Autodesk Fusion 360 part; units mm, degrees
(part 10 of 40)
  spline S57 degree 5 poles (181.0205, 97.4897) (181.0048, 97.4632) (180.9726, 97.4105) (180.9223, 97.3328) (180.8513, 97.2319) (180.7572, 97.1094) (180.6593, 96.9894) (180.5591, 96.8711) (180.4576, 96.7536) (180.3553, 96.6366) (180.252, 96.5203) (180.1476, 96.4049) (180.0417, 96.2906) (179.9339, 96.1776) (179.8243, 96.066) (179.713, 95.9556) (179.6004, 95.8463) (179.4865, 95.7378) (179.3717, 95.6302) (179.256, 95.5233) (179.1393, 95.4172) (179.0215, 95.3119) (178.9028, 95.2074) (178.7829, 95.1039) (178.662, 95.0012) (178.5401, 94.8993) (178.4172, 94.7983) (178.2934, 94.698) (178.1687, 94.5985) (178.0432, 94.4997) (177.9169, 94.4016) (177.7897, 94.3043) (177.6617, 94.2077) (177.5329, 94.1119) (177.4032, 94.0168) (177.2728, 93.9224) (177.1415, 93.8288) (177.0096, 93.7358) (176.8768, 93.6436) (176.7434, 93.552) (176.6092, 93.4612) (176.4743, 93.371) (176.3387, 93.2815) (176.2025, 93.1927) (176.0655, 93.1045) (175.9278, 93.0171) (175.7895, 92.9303) (175.6505, 92.8442) (175.5109, 92.7587) (175.3706, 92.6739) (175.2297, 92.5898) (175.0882, 92.5063) (174.946, 92.4235) (174.8032, 92.3413) (174.6599, 92.2597) (174.5159, 92.1788) (174.3713, 92.0986) (174.2262, 92.019) (174.0805, 91.94) (173.9342, 91.8617) (173.7873, 91.784) (173.6399, 91.7069) (173.4919, 91.6305) (173.3434, 91.5547) (173.1943, 91.4795) (173.0447, 91.405) (172.8946, 91.331) (172.7439, 91.2577) (172.5927, 91.1851) (172.4411, 91.113) (172.2889, 91.0416) (172.1667, 90.9849) (172.0748, 90.9427) (172.0135, 90.9147) (171.9828, 90.9007) knots 0 0 0 0 0 0 0.01428571 0.02857143 0.04285714 0.05714286 0.07142857 0.08571429 0.1 0.11428571 0.12857143 0.14285714 0.15714286 0.17142857 0.18571429 0.2 0.21428571 0.22857143 0.24285714 0.25714286 0.27142857 0.28571429 0.3 0.31428571 0.32857143 0.34285714 0.35714286 0.37142857 0.38571429 0.4 0.41428571 0.42857143 0.44285714 0.45714286 0.47142857 0.48571429 0.5 0.51428571 0.52857143 0.54285714 0.55714286 0.57142857 0.58571429 0.6 0.61428571 0.62857143 0.64285714 0.65714286 0.67142857 0.68571429 0.7 0.71428571 0.72857143 0.74285714 0.75714286 0.77142857 0.78571429 0.8 0.81428571 0.82857143 0.84285714 0.85714286 0.87142857 0.88571429 0.9 0.91428571 0.92857143 0.94285714 0.95714286 0.97142857 0.98571429 1 1 1 1 1 1
  line L4287 (181.0205, 97.4897) -> (181.0048, 97.4632) construction
  line L4288 (181.0048, 97.4632) -> (180.9726, 97.4105) construction
  line L4289 (180.9726, 97.4105) -> (180.9223, 97.3328) construction
  line L4290 (180.9223, 97.3328) -> (180.8513, 97.2319) construction
  line L4291 (180.8513, 97.2319) -> (180.7572, 97.1094) construction
  line L4292 (180.7572, 97.1094) -> (180.6593, 96.9894) construction
  line L4293 (180.6593, 96.9894) -> (180.5591, 96.8711) construction
  line L4294 (180.5591, 96.8711) -> (180.4576, 96.7536) construction
  line L4295 (180.4576, 96.7536) -> (180.3553, 96.6366) construction
  line L4296 (180.3553, 96.6366) -> (180.252, 96.5203) construction
  line L4297 (180.252, 96.5203) -> (180.1476, 96.4049) construction
  line L4298 (180.1476, 96.4049) -> (180.0417, 96.2906) construction
  line L4299 (180.0417, 96.2906) -> (179.9339, 96.1776) construction
  line L4300 (179.9339, 96.1776) -> (179.8243, 96.066) construction
  line L4301 (179.8243, 96.066) -> (179.713, 95.9556) construction
  line L4302 (179.713, 95.9556) -> (179.6004, 95.8463) construction
  line L4303 (179.6004, 95.8463) -> (179.4865, 95.7378) construction
  line L4304 (179.4865, 95.7378) -> (179.3717, 95.6302) construction
  line L4305 (179.3717, 95.6302) -> (179.256, 95.5233) construction
  line L4306 (179.256, 95.5233) -> (179.1393, 95.4172) construction
  line L4307 (179.1393, 95.4172) -> (179.0215, 95.3119) construction
  line L4308 (179.0215, 95.3119) -> (178.9028, 95.2074) construction
  line L4309 (178.9028, 95.2074) -> (178.7829, 95.1039) construction
  line L4310 (178.7829, 95.1039) -> (178.662, 95.0012) construction
  line L4311 (178.662, 95.0012) -> (178.5401, 94.8993) construction
  line L4312 (178.5401, 94.8993) -> (178.4172, 94.7983) construction
  line L4313 (178.4172, 94.7983) -> (178.2934, 94.698) construction
  line L4314 (178.2934, 94.698) -> (178.1687, 94.5985) construction
  line L4315 (178.1687, 94.5985) -> (178.0432, 94.4997) construction
  line L4316 (178.0432, 94.4997) -> (177.9169, 94.4016) construction
  line L4317 (177.9169, 94.4016) -> (177.7897, 94.3043) construction
  line L4318 (177.7897, 94.3043) -> (177.6617, 94.2077) construction
  line L4319 (177.6617, 94.2077) -> (177.5329, 94.1119) construction
  line L4320 (177.5329, 94.1119) -> (177.4032, 94.0168) construction
  line L4321 (177.4032, 94.0168) -> (177.2728, 93.9224) construction
  line L4322 (177.2728, 93.9224) -> (177.1415, 93.8288) construction
  line L4323 (177.1415, 93.8288) -> (177.0096, 93.7358) construction
  line L4324 (177.0096, 93.7358) -> (176.8768, 93.6436) construction
  line L4325 (176.8768, 93.6436) -> (176.7434, 93.552) construction
  line L4326 (176.7434, 93.552) -> (176.6092, 93.4612) construction
  line L4327 (176.6092, 93.4612) -> (176.4743, 93.371) construction
  line L4328 (176.4743, 93.371) -> (176.3387, 93.2815) construction
  line L4329 (176.3387, 93.2815) -> (176.2025, 93.1927) construction
  line L4330 (176.2025, 93.1927) -> (176.0655, 93.1045) construction
  line L4331 (176.0655, 93.1045) -> (175.9278, 93.0171) construction
  line L4332 (175.9278, 93.0171) -> (175.7895, 92.9303) construction
  line L4333 (175.7895, 92.9303) -> (175.6505, 92.8442) construction
  line L4334 (175.6505, 92.8442) -> (175.5109, 92.7587) construction
  line L4335 (175.5109, 92.7587) -> (175.3706, 92.6739) construction
  line L4336 (175.3706, 92.6739) -> (175.2297, 92.5898) construction
  line L4337 (175.2297, 92.5898) -> (175.0882, 92.5063) construction
  line L4338 (175.0882, 92.5063) -> (174.946, 92.4235) construction
  line L4339 (174.946, 92.4235) -> (174.8032, 92.3413) construction
  line L4340 (174.8032, 92.3413) -> (174.6599, 92.2597) construction
  line L4341 (174.6599, 92.2597) -> (174.5159, 92.1788) construction
  line L4342 (174.5159, 92.1788) -> (174.3713, 92.0986) construction
  line L4343 (174.3713, 92.0986) -> (174.2262, 92.019) construction
  line L4344 (174.2262, 92.019) -> (174.0805, 91.94) construction
  line L4345 (174.0805, 91.94) -> (173.9342, 91.8617) construction
  line L4346 (173.9342, 91.8617) -> (173.7873, 91.784) construction
  line L4347 (173.7873, 91.784) -> (173.6399, 91.7069) construction
  line L4348 (173.6399, 91.7069) -> (173.4919, 91.6305) construction
  line L4349 (173.4919, 91.6305) -> (173.3434, 91.5547) construction
  line L4350 (173.3434, 91.5547) -> (173.1943, 91.4795) construction
  line L4351 (173.1943, 91.4795) -> (173.0447, 91.405) construction
  line L4352 (173.0447, 91.405) -> (172.8946, 91.331) construction
  line L4353 (172.8946, 91.331) -> (172.7439, 91.2577) construction
  line L4354 (172.7439, 91.2577) -> (172.5927, 91.1851) construction
  line L4355 (172.5927, 91.1851) -> (172.4411, 91.113) construction
  line L4356 (172.4411, 91.113) -> (172.2889, 91.0416) construction
  line L4357 (172.2889, 91.0416) -> (172.1667, 90.9849) construction
  line L4358 (172.1667, 90.9849) -> (172.0748, 90.9427) construction
  line L4359 (172.0748, 90.9427) -> (172.0135, 90.9147) construction
  line L4360 (172.0135, 90.9147) -> (171.9828, 90.9007) construction
  spline S58 degree 5 poles (171.8057, 104.1847) (171.7853, 104.1615) (171.7452, 104.1146) (171.6869, 104.0427) (171.6128, 103.944) (171.5254, 103.8167) (171.4416, 103.6865) (171.36, 103.5546) (171.2796, 103.4218) (171.2, 103.2883) (171.1213, 103.1542) (171.0437, 103.0193) (170.9678, 102.8832) (170.8937, 102.7457) (170.8214, 102.607) (170.7507, 102.4671) (170.6816, 102.3262) (170.6136, 102.1844) (170.5467, 102.0419) (170.4808, 101.8988) (170.416, 101.755) (170.3522, 101.6105) (170.2896, 101.4653) (170.2281, 101.3193) (170.1678, 101.1726) (170.1086, 101.0251) (170.0505, 100.877) (169.9934, 100.7283) (169.9373, 100.579) (169.8821, 100.4291) (169.8279, 100.2786) (169.7746, 100.1276) (169.7223, 99.976) (169.671, 99.8239) (169.6206, 99.6712) (169.5712, 99.518) (169.5226, 99.3642) (169.475, 99.21) (169.4283, 99.0553) (169.3825, 98.9001) (169.3375, 98.7444) (169.2934, 98.5882) (169.2502, 98.4316) (169.2079, 98.2745) (169.1664, 98.117) (169.1257, 97.9591) (169.0859, 97.8007) (169.047, 97.6419) (169.0089, 97.4827) (168.9716, 97.3231) (168.9351, 97.1631) (168.8994, 97.0027) (168.8646, 96.8419) (168.8305, 96.6807) (168.7973, 96.5191) (168.7648, 96.3572) (168.7332, 96.1949) (168.7023, 96.0323) (168.6723, 95.8693) (168.643, 95.706) (168.6145, 95.5423) (168.5867, 95.3783) (168.5597, 95.2139) (168.5336, 95.0492) (168.5081, 94.8842) (168.4834, 94.7189) (168.4595, 94.5533) (168.4364, 94.3874) (168.414, 94.2211) (168.3923, 94.0546) (168.3714, 93.8878) (168.3553, 93.7541) (168.3435, 93.6537) (168.3358, 93.5867) (168.332, 93.5531) knots 0 0 0 0 0 0 0.01428571 0.02857143 0.04285714 0.05714286 0.07142857 0.08571429 0.1 0.11428571 0.12857143 0.14285714 0.15714286 0.17142857 0.18571429 0.2 0.21428571 0.22857143 0.24285714 0.25714286 0.27142857 0.28571429 0.3 0.31428571 0.32857143 0.34285714 0.35714286 0.37142857 0.38571429 0.4 0.41428571 0.42857143 0.44285714 0.45714286 0.47142857 0.48571429 0.5 0.51428571 0.52857143 0.54285714 0.55714286 0.57142857 0.58571429 0.6 0.61428571 0.62857143 0.64285714 0.65714286 0.67142857 0.68571429 0.7 0.71428571 0.72857143 0.74285714 0.75714286 0.77142857 0.78571429 0.8 0.81428571 0.82857143 0.84285714 0.85714286 0.87142857 0.88571429 0.9 0.91428571 0.92857143 0.94285714 0.95714286 0.97142857 0.98571429 1 1 1 1 1 1
  line L4361 (171.8057, 104.1847) -> (171.7853, 104.1615) construction
  line L4362 (171.7853, 104.1615) -> (171.7452, 104.1146) construction
  line L4363 (171.7452, 104.1146) -> (171.6869, 104.0427) construction
  line L4364 (171.6869, 104.0427) -> (171.6128, 103.944) construction
  line L4365 (171.6128, 103.944) -> (171.5254, 103.8167) construction
  line L4366 (171.5254, 103.8167) -> (171.4416, 103.6865) construction
  line L4367 (171.4416, 103.6865) -> (171.36, 103.5546) construction
  line L4368 (171.36, 103.5546) -> (171.2796, 103.4218) construction
  line L4369 (171.2796, 103.4218) -> (171.2, 103.2883) construction
  line L4370 (171.2, 103.2883) -> (171.1213, 103.1542) construction
  line L4371 (171.1213, 103.1542) -> (171.0437, 103.0193) construction
  line L4372 (171.0437, 103.0193) -> (170.9678, 102.8832) construction
  line L4373 (170.9678, 102.8832) -> (170.8937, 102.7457) construction
  line L4374 (170.8937, 102.7457) -> (170.8214, 102.607) construction
  line L4375 (170.8214, 102.607) -> (170.7507, 102.4671) construction
  line L4376 (170.7507, 102.4671) -> (170.6816, 102.3262) construction
  line L4377 (170.6816, 102.3262) -> (170.6136, 102.1844) construction
  line L4378 (170.6136, 102.1844) -> (170.5467, 102.0419) construction
  line L4379 (170.5467, 102.0419) -> (170.4808, 101.8988) construction
  line L4380 (170.4808, 101.8988) -> (170.416, 101.755) construction
  line L4381 (170.416, 101.755) -> (170.3522, 101.6105) construction
  line L4382 (170.3522, 101.6105) -> (170.2896, 101.4653) construction
  line L4383 (170.2896, 101.4653) -> (170.2281, 101.3193) construction
  line L4384 (170.2281, 101.3193) -> (170.1678, 101.1726) construction
  line L4385 (170.1678, 101.1726) -> (170.1086, 101.0251) construction
  line L4386 (170.1086, 101.0251) -> (170.0505, 100.877) construction
  line L4387 (170.0505, 100.877) -> (169.9934, 100.7283) construction
  line L4388 (169.9934, 100.7283) -> (169.9373, 100.579) construction
  line L4389 (169.9373, 100.579) -> (169.8821, 100.4291) construction
  line L4390 (169.8821, 100.4291) -> (169.8279, 100.2786) construction
  line L4391 (169.8279, 100.2786) -> (169.7746, 100.1276) construction
  line L4392 (169.7746, 100.1276) -> (169.7223, 99.976) construction
  line L4393 (169.7223, 99.976) -> (169.671, 99.8239) construction
  line L4394 (169.671, 99.8239) -> (169.6206, 99.6712) construction
  line L4395 (169.6206, 99.6712) -> (169.5712, 99.518) construction
  line L4396 (169.5712, 99.518) -> (169.5226, 99.3642) construction
  line L4397 (169.5226, 99.3642) -> (169.475, 99.21) construction
  line L4398 (169.475, 99.21) -> (169.4283, 99.0553) construction
  line L4399 (169.4283, 99.0553) -> (169.3825, 98.9001) construction
  line L4400 (169.3825, 98.9001) -> (169.3375, 98.7444) construction
  line L4401 (169.3375, 98.7444) -> (169.2934, 98.5882) construction
  line L4402 (169.2934, 98.5882) -> (169.2502, 98.4316) construction
  line L4403 (169.2502, 98.4316) -> (169.2079, 98.2745) construction
  line L4404 (169.2079, 98.2745) -> (169.1664, 98.117) construction
  line L4405 (169.1664, 98.117) -> (169.1257, 97.9591) construction
  line L4406 (169.1257, 97.9591) -> (169.0859, 97.8007) construction
  line L4407 (169.0859, 97.8007) -> (169.047, 97.6419) construction
  line L4408 (169.047, 97.6419) -> (169.0089, 97.4827) construction
  line L4409 (169.0089, 97.4827) -> (168.9716, 97.3231) construction
  line L4410 (168.9716, 97.3231) -> (168.9351, 97.1631) construction
  line L4411 (168.9351, 97.1631) -> (168.8994, 97.0027) construction
  line L4412 (168.8994, 97.0027) -> (168.8646, 96.8419) construction
  line L4413 (168.8646, 96.8419) -> (168.8305, 96.6807) construction
  line L4414 (168.8305, 96.6807) -> (168.7973, 96.5191) construction
  line L4415 (168.7973, 96.5191) -> (168.7648, 96.3572) construction
  line L4416 (168.7648, 96.3572) -> (168.7332, 96.1949) construction
  line L4417 (168.7332, 96.1949) -> (168.7023, 96.0323) construction
  line L4418 (168.7023, 96.0323) -> (168.6723, 95.8693) construction
  line L4419 (168.6723, 95.8693) -> (168.643, 95.706) construction
  line L4420 (168.643, 95.706) -> (168.6145, 95.5423) construction
  line L4421 (168.6145, 95.5423) -> (168.5867, 95.3783) construction
  line L4422 (168.5867, 95.3783) -> (168.5597, 95.2139) construction
  line L4423 (168.5597, 95.2139) -> (168.5336, 95.0492) construction
  line L4424 (168.5336, 95.0492) -> (168.5081, 94.8842) construction
  line L4425 (168.5081, 94.8842) -> (168.4834, 94.7189) construction
  line L4426 (168.4834, 94.7189) -> (168.4595, 94.5533) construction
  line L4427 (168.4595, 94.5533) -> (168.4364, 94.3874) construction
  line L4428 (168.4364, 94.3874) -> (168.414, 94.2211) construction
  line L4429 (168.414, 94.2211) -> (168.3923, 94.0546) construction
  line L4430 (168.3923, 94.0546) -> (168.3714, 93.8878) construction
  line L4431 (168.3714, 93.8878) -> (168.3553, 93.7541) construction
  line L4432 (168.3553, 93.7541) -> (168.3435, 93.6537) construction
  line L4433 (168.3435, 93.6537) -> (168.3358, 93.5867) construction
  line L4434 (168.3358, 93.5867) -> (168.332, 93.5531) construction
  spline S59 degree 5 poles (268.1665, 125.8052) (268.1948, 125.7929) (268.2518, 125.7692) (268.3382, 125.736) (268.4549, 125.6961) (268.6031, 125.6522) (268.7528, 125.6127) (268.9034, 125.5759) (269.0546, 125.5405) (269.2061, 125.506) (269.358, 125.4726) (269.5103, 125.4406) (269.6632, 125.4104) (269.8168, 125.3824) (269.9711, 125.3565) (270.126, 125.3326) (270.2814, 125.3103) (270.4372, 125.2895) (270.5934, 125.2699) (270.7499, 125.2515) (270.9067, 125.2342) (271.0638, 125.2182) (271.2213, 125.2035) (271.3791, 125.1902) (271.5373, 125.1782) (271.6958, 125.1675) (271.8546, 125.158) (272.0137, 125.1496) (272.1731, 125.1423) (272.3327, 125.1362) (272.4925, 125.1311) (272.6526, 125.1271) (272.8129, 125.1243) (272.9735, 125.1224) (273.1343, 125.1217) (273.2953, 125.122) (273.4565, 125.1234) (273.6179, 125.1258) (273.7795, 125.1292) (273.9413, 125.1335) (274.1032, 125.1389) (274.2654, 125.1452) (274.4277, 125.1525) (274.5901, 125.1608) (274.7527, 125.17) (274.9155, 125.1801) (275.0784, 125.1912) (275.2415, 125.2033) (275.4047, 125.2162) (275.568, 125.23) (275.7315, 125.2448) (275.8951, 125.2604) (276.0588, 125.277) (276.2226, 125.2944) (276.3865, 125.3127) (276.5505, 125.3319) (276.7146, 125.352) (276.8788, 125.3729) (277.0431, 125.3946) (277.2075, 125.4172) (277.372, 125.4407) (277.5366, 125.465) (277.7012, 125.4902) (277.866, 125.5161) (278.0307, 125.5429) (278.1956, 125.5706) (278.3605, 125.599) (278.5255, 125.6282) (278.6905, 125.6583) (278.8556, 125.6892) (279.0207, 125.7208) (279.1528, 125.7468) (279.2519, 125.7666) (279.318, 125.78) (279.3511, 125.7868) knots 0 0 0 0 0 0 0.01428571 0.02857143 0.04285714 0.05714286 0.07142857 0.08571429 0.1 0.11428571 0.12857143 0.14285714 0.15714286 0.17142857 0.18571429 0.2 0.21428571 0.22857143 0.24285714 0.25714286 0.27142857 0.28571429 0.3 0.31428571 0.32857143 0.34285714 0.35714286 0.37142857 0.38571429 0.4 0.41428571 0.42857143 0.44285714 0.45714286 0.47142857 0.48571429 0.5 0.51428571 0.52857143 0.54285714 0.55714286 0.57142857 0.58571429 0.6 0.61428571 0.62857143 0.64285714 0.65714286 0.67142857 0.68571429 0.7 0.71428571 0.72857143 0.74285714 0.75714286 0.77142857 0.78571429 0.8 0.81428571 0.82857143 0.84285714 0.85714286 0.87142857 0.88571429 0.9 0.91428571 0.92857143 0.94285714 0.95714286 0.97142857 0.98571429 1 1 1 1 1 1
  line L4435 (268.1665, 125.8052) -> (268.1948, 125.7929) construction
  line L4436 (268.1948, 125.7929) -> (268.2518, 125.7692) construction
  line L4437 (268.2518, 125.7692) -> (268.3382, 125.736) construction
  line L4438 (268.3382, 125.736) -> (268.4549, 125.6961) construction
  line L4439 (268.4549, 125.6961) -> (268.6031, 125.6522) construction
  line L4440 (268.6031, 125.6522) -> (268.7528, 125.6127) construction
  line L4441 (268.7528, 125.6127) -> (268.9034, 125.5759) construction
  line L4442 (268.9034, 125.5759) -> (269.0546, 125.5405) construction
  line L4443 (269.0546, 125.5405) -> (269.2061, 125.506) construction
  line L4444 (269.2061, 125.506) -> (269.358, 125.4726) construction
  line L4445 (269.358, 125.4726) -> (269.5103, 125.4406) construction
  line L4446 (269.5103, 125.4406) -> (269.6632, 125.4104) construction
  line L4447 (269.6632, 125.4104) -> (269.8168, 125.3824) construction
  line L4448 (269.8168, 125.3824) -> (269.9711, 125.3565) construction
  line L4449 (269.9711, 125.3565) -> (270.126, 125.3326) construction
  line L4450 (270.126, 125.3326) -> (270.2814, 125.3103) construction
  line L4451 (270.2814, 125.3103) -> (270.4372, 125.2895) construction
  line L4452 (270.4372, 125.2895) -> (270.5934, 125.2699) construction
  line L4453 (270.5934, 125.2699) -> (270.7499, 125.2515) construction
  line L4454 (270.7499, 125.2515) -> (270.9067, 125.2342) construction
  line L4455 (270.9067, 125.2342) -> (271.0638, 125.2182) construction
  line L4456 (271.0638, 125.2182) -> (271.2213, 125.2035) construction
  line L4457 (271.2213, 125.2035) -> (271.3791, 125.1902) construction
  line L4458 (271.3791, 125.1902) -> (271.5373, 125.1782) construction
  line L4459 (271.5373, 125.1782) -> (271.6958, 125.1675) construction
  line L4460 (271.6958, 125.1675) -> (271.8546, 125.158) construction
  line L4461 (271.8546, 125.158) -> (272.0137, 125.1496) construction
  line L4462 (272.0137, 125.1496) -> (272.1731, 125.1423) construction
  line L4463 (272.1731, 125.1423) -> (272.3327, 125.1362) construction
  line L4464 (272.3327, 125.1362) -> (272.4925, 125.1311) construction
  line L4465 (272.4925, 125.1311) -> (272.6526, 125.1271) construction
  line L4466 (272.6526, 125.1271) -> (272.8129, 125.1243) construction
  line L4467 (272.8129, 125.1243) -> (272.9735, 125.1224) construction
  line L4468 (272.9735, 125.1224) -> (273.1343, 125.1217) construction
  line L4469 (273.1343, 125.1217) -> (273.2953, 125.122) construction
  line L4470 (273.2953, 125.122) -> (273.4565, 125.1234) construction
  line L4471 (273.4565, 125.1234) -> (273.6179, 125.1258) construction
  line L4472 (273.6179, 125.1258) -> (273.7795, 125.1292) construction
  line L4473 (273.7795, 125.1292) -> (273.9413, 125.1335) construction
  line L4474 (273.9413, 125.1335) -> (274.1032, 125.1389) construction
  line L4475 (274.1032, 125.1389) -> (274.2654, 125.1452) construction
  line L4476 (274.2654, 125.1452) -> (274.4277, 125.1525) construction
  line L4477 (274.4277, 125.1525) -> (274.5901, 125.1608) construction
  line L4478 (274.5901, 125.1608) -> (274.7527, 125.17) construction
  line L4479 (274.7527, 125.17) -> (274.9155, 125.1801) construction
  line L4480 (274.9155, 125.1801) -> (275.0784, 125.1912) construction
  line L4481 (275.0784, 125.1912) -> (275.2415, 125.2033) construction
  line L4482 (275.2415, 125.2033) -> (275.4047, 125.2162) construction
  line L4483 (275.4047, 125.2162) -> (275.568, 125.23) construction
  line L4484 (275.568, 125.23) -> (275.7315, 125.2448) construction
  line L4485 (275.7315, 125.2448) -> (275.8951, 125.2604) construction
  line L4486 (275.8951, 125.2604) -> (276.0588, 125.277) construction
  line L4487 (276.0588, 125.277) -> (276.2226, 125.2944) construction
  line L4488 (276.2226, 125.2944) -> (276.3865, 125.3127) construction
  line L4489 (276.3865, 125.3127) -> (276.5505, 125.3319) construction
  line L4490 (276.5505, 125.3319) -> (276.7146, 125.352) construction
  line L4491 (276.7146, 125.352) -> (276.8788, 125.3729) construction
  line L4492 (276.8788, 125.3729) -> (277.0431, 125.3946) construction
  line L4493 (277.0431, 125.3946) -> (277.2075, 125.4172) construction
  line L4494 (277.2075, 125.4172) -> (277.372, 125.4407) construction
  line L4495 (277.372, 125.4407) -> (277.5366, 125.465) construction
  line L4496 (277.5366, 125.465) -> (277.7012, 125.4902) construction
  line L4497 (277.7012, 125.4902) -> (277.866, 125.5161) construction
  line L4498 (277.866, 125.5161) -> (278.0307, 125.5429) construction
  line L4499 (278.0307, 125.5429) -> (278.1956, 125.5706) construction
  line L4500 (278.1956, 125.5706) -> (278.3605, 125.599) construction
  line L4501 (278.3605, 125.599) -> (278.5255, 125.6282) construction
  line L4502 (278.5255, 125.6282) -> (278.6905, 125.6583) construction
  line L4503 (278.6905, 125.6583) -> (278.8556, 125.6892) construction
  line L4504 (278.8556, 125.6892) -> (279.0207, 125.7208) construction
  line L4505 (279.0207, 125.7208) -> (279.1528, 125.7468) construction
  line L4506 (279.1528, 125.7468) -> (279.2519, 125.7666) construction
  line L4507 (279.2519, 125.7666) -> (279.318, 125.78) construction
  line L4508 (279.318, 125.78) -> (279.3511, 125.7868) construction
  spline S60 degree 5 poles (264.6423, 118.8885) (264.6688, 118.8728) (264.7215, 118.8406) (264.7992, 118.7903) (264.9001, 118.7193) (265.0226, 118.6252) (265.1426, 118.5273) (265.2609, 118.4271) (265.3784, 118.3256) (265.4954, 118.2233) (265.6117, 118.12) (265.7271, 118.0156) (265.8414, 117.9097) (265.9544, 117.8019) (266.066, 117.6923) (266.1764, 117.581) (266.2857, 117.4684) (266.3942, 117.3545) (266.5018, 117.2397) (266.6087, 117.124) (266.7148, 117.0073) (266.8201, 116.8895) (266.9246, 116.7708) (267.0281, 116.6509) (267.1308, 116.53) (267.2327, 116.4081) (267.3337, 116.2852) (267.434, 116.1614) (267.5335, 116.0367) (267.6323, 115.9112) (267.7304, 115.7849) (267.8277, 115.6577) (267.9243, 115.5297) (268.0201, 115.4009) (268.1152, 115.2712) (268.2096, 115.1408) (268.3032, 115.0095) (268.3962, 114.8776) (268.4884, 114.7448) (268.58, 114.6114) (268.6708, 114.4772) (268.761, 114.3423) (268.8505, 114.2067) (268.9393, 114.0705) (269.0275, 113.9335) (269.1149, 113.7958) (269.2017, 113.6575) (269.2878, 113.5185) (269.3733, 113.3789) (269.4581, 113.2386) (269.5422, 113.0977) (269.6257, 112.9562) (269.7085, 112.814) (269.7907, 112.6712) (269.8723, 112.5279) (269.9532, 112.3839) (270.0334, 112.2393) (270.113, 112.0942) (270.192, 111.9485) (270.2703, 111.8022) (270.348, 111.6553) (270.4251, 111.5079) (270.5015, 111.3599) (270.5773, 111.2114) (270.6525, 111.0623) (270.727, 110.9127) (270.801, 110.7626) (270.8743, 110.6119) (270.9469, 110.4607) (271.019, 110.3091) (271.0904, 110.1569) (271.1471, 110.0347) (271.1893, 109.9428) (271.2173, 109.8815) (271.2313, 109.8508) knots 0 0 0 0 0 0 0.01428571 0.02857143 0.04285714 0.05714286 0.07142857 0.08571429 0.1 0.11428571 0.12857143 0.14285714 0.15714286 0.17142857 0.18571429 0.2 0.21428571 0.22857143 0.24285714 0.25714286 0.27142857 0.28571429 0.3 0.31428571 0.32857143 0.34285714 0.35714286 0.37142857 0.38571429 0.4 0.41428571 0.42857143 0.44285714 0.45714286 0.47142857 0.48571429 0.5 0.51428571 0.52857143 0.54285714 0.55714286 0.57142857 0.58571429 0.6 0.61428571 0.62857143 0.64285714 0.65714286 0.67142857 0.68571429 0.7 0.71428571 0.72857143 0.74285714 0.75714286 0.77142857 0.78571429 0.8 0.81428571 0.82857143 0.84285714 0.85714286 0.87142857 0.88571429 0.9 0.91428571 0.92857143 0.94285714 0.95714286 0.97142857 0.98571429 1 1 1 1 1 1
  line L4509 (264.6423, 118.8885) -> (264.6688, 118.8728) construction
  line L4510 (264.6688, 118.8728) -> (264.7215, 118.8406) construction
  line L4511 (264.7215, 118.8406) -> (264.7992, 118.7903) construction
  line L4512 (264.7992, 118.7903) -> (264.9001, 118.7193) construction
  line L4513 (264.9001, 118.7193) -> (265.0226, 118.6252) construction
  line L4514 (265.0226, 118.6252) -> (265.1426, 118.5273) construction
  line L4515 (265.1426, 118.5273) -> (265.2609, 118.4271) construction
  line L4516 (265.2609, 118.4271) -> (265.3784, 118.3256) construction
  line L4517 (265.3784, 118.3256) -> (265.4954, 118.2233) construction
  line L4518 (265.4954, 118.2233) -> (265.6117, 118.12) construction
  line L4519 (265.6117, 118.12) -> (265.7271, 118.0156) construction
  line L4520 (265.7271, 118.0156) -> (265.8414, 117.9097) construction
  line L4521 (265.8414, 117.9097) -> (265.9544, 117.8019) construction
  line L4522 (265.9544, 117.8019) -> (266.066, 117.6923) construction
  line L4523 (266.066, 117.6923) -> (266.1764, 117.581) construction
  line L4524 (266.1764, 117.581) -> (266.2857, 117.4684) construction
  line L4525 (266.2857, 117.4684) -> (266.3942, 117.3545) construction
  line L4526 (266.3942, 117.3545) -> (266.5018, 117.2397) construction
  line L4527 (266.5018, 117.2397) -> (266.6087, 117.124) construction
  line L4528 (266.6087, 117.124) -> (266.7148, 117.0073) construction
  line L4529 (266.7148, 117.0073) -> (266.8201, 116.8895) construction
  line L4530 (266.8201, 116.8895) -> (266.9246, 116.7708) construction
  line L4531 (266.9246, 116.7708) -> (267.0281, 116.6509) construction
  line L4532 (267.0281, 116.6509) -> (267.1308, 116.53) construction
  line L4533 (267.1308, 116.53) -> (267.2327, 116.4081) construction
  line L4534 (267.2327, 116.4081) -> (267.3337, 116.2852) construction
  line L4535 (267.3337, 116.2852) -> (267.434, 116.1614) construction
  line L4536 (267.434, 116.1614) -> (267.5335, 116.0367) construction
  line L4537 (267.5335, 116.0367) -> (267.6323, 115.9112) construction
  line L4538 (267.6323, 115.9112) -> (267.7304, 115.7849) construction
  line L4539 (267.7304, 115.7849) -> (267.8277, 115.6577) construction
  line L4540 (267.8277, 115.6577) -> (267.9243, 115.5297) construction
  line L4541 (267.9243, 115.5297) -> (268.0201, 115.4009) construction
  line L4542 (268.0201, 115.4009) -> (268.1152, 115.2712) construction
  line L4543 (268.1152, 115.2712) -> (268.2096, 115.1408) construction
  line L4544 (268.2096, 115.1408) -> (268.3032, 115.0095) construction
  line L4545 (268.3032, 115.0095) -> (268.3962, 114.8776) construction
  line L4546 (268.3962, 114.8776) -> (268.4884, 114.7448) construction
  line L4547 (268.4884, 114.7448) -> (268.58, 114.6114) construction
  line L4548 (268.58, 114.6114) -> (268.6708, 114.4772) construction
  line L4549 (268.6708, 114.4772) -> (268.761, 114.3423) construction
  line L4550 (268.761, 114.3423) -> (268.8505, 114.2067) construction
  line L4551 (268.8505, 114.2067) -> (268.9393, 114.0705) construction
  line L4552 (268.9393, 114.0705) -> (269.0275, 113.9335) construction
  line L4553 (269.0275, 113.9335) -> (269.1149, 113.7958) construction
  line L4554 (269.1149, 113.7958) -> (269.2017, 113.6575) construction
  line L4555 (269.2017, 113.6575) -> (269.2878, 113.5185) construction
  line L4556 (269.2878, 113.5185) -> (269.3733, 113.3789) construction
  line L4557 (269.3733, 113.3789) -> (269.4581, 113.2386) construction
  line L4558 (269.4581, 113.2386) -> (269.5422, 113.0977) construction
  line L4559 (269.5422, 113.0977) -> (269.6257, 112.9562) construction
  line L4560 (269.6257, 112.9562) -> (269.7085, 112.814) construction
  line L4561 (269.7085, 112.814) -> (269.7907, 112.6712) construction
  line L4562 (269.7907, 112.6712) -> (269.8723, 112.5279) construction
  line L4563 (269.8723, 112.5279) -> (269.9532, 112.3839) construction
  line L4564 (269.9532, 112.3839) -> (270.0334, 112.2393) construction
  line L4565 (270.0334, 112.2393) -> (270.113, 112.0942) construction
  line L4566 (270.113, 112.0942) -> (270.192, 111.9485) construction
  line L4567 (270.192, 111.9485) -> (270.2703, 111.8022) construction
  line L4568 (270.2703, 111.8022) -> (270.348, 111.6553) construction
  line L4569 (270.348, 111.6553) -> (270.4251, 111.5079) construction
  line L4570 (270.4251, 111.5079) -> (270.5015, 111.3599) construction
  line L4571 (270.5015, 111.3599) -> (270.5773, 111.2114) construction
  line L4572 (270.5773, 111.2114) -> (270.6525, 111.0623) construction
  line L4573 (270.6525, 111.0623) -> (270.727, 110.9127) construction
  line L4574 (270.727, 110.9127) -> (270.801, 110.7626) construction
  line L4575 (270.801, 110.7626) -> (270.8743, 110.6119) construction
  line L4576 (270.8743, 110.6119) -> (270.9469, 110.4607) construction
  line L4577 (270.9469, 110.4607) -> (271.019, 110.3091) construction
  line L4578 (271.019, 110.3091) -> (271.0904, 110.1569) construction
  line L4579 (271.0904, 110.1569) -> (271.1471, 110.0347) construction
  line L4580 (271.1471, 110.0347) -> (271.1893, 109.9428) construction
  line L4581 (271.1893, 109.9428) -> (271.2173, 109.8815) construction
  line L4582 (271.2173, 109.8815) -> (271.2313, 109.8508) construction
  spline S61 degree 5 poles (264.6423, 118.8885) (264.6688, 118.8728) (264.7215, 118.8406) (264.7992, 118.7903) (264.9001, 118.7193) (265.0226, 118.6252) (265.1426, 118.5273) (265.2609, 118.4271) (265.3784, 118.3256) (265.4954, 118.2233) (265.6117, 118.12) (265.7271, 118.0156) (265.8414, 117.9097) (265.9544, 117.8019) (266.066, 117.6923) (266.1764, 117.581) (266.2857, 117.4684) (266.3942, 117.3545) (266.5018, 117.2397) (266.6087, 117.124) (266.7148, 117.0073) (266.8201, 116.8895) (266.9246, 116.7708) (267.0281, 116.6509) (267.1308, 116.53) (267.2327, 116.4081) (267.3337, 116.2852) (267.434, 116.1614) (267.5335, 116.0367) (267.6323, 115.9112) (267.7304, 115.7849) (267.8277, 115.6577) (267.9243, 115.5297) (268.0201, 115.4009) (268.1152, 115.2712) (268.2096, 115.1408) (268.3032, 115.0095) (268.3962, 114.8776) (268.4884, 114.7448) (268.58, 114.6114) (268.6708, 114.4772) (268.761, 114.3423) (268.8505, 114.2067) (268.9393, 114.0705) (269.0275, 113.9335) (269.1149, 113.7958) (269.2017, 113.6575) (269.2878, 113.5185) (269.3733, 113.3789) (269.4581, 113.2386) (269.5422, 113.0977) (269.6257, 112.9562) (269.7085, 112.814) (269.7907, 112.6712) (269.8723, 112.5279) (269.9532, 112.3839) (270.0334, 112.2393) (270.113, 112.0942) (270.192, 111.9485) (270.2703, 111.8022) (270.348, 111.6553) (270.4251, 111.5079) (270.5015, 111.3599) (270.5773, 111.2114) (270.6525, 111.0623) (270.727, 110.9127) (270.801, 110.7626) (270.8743, 110.6119) (270.9469, 110.4607) (271.019, 110.3091) (271.0904, 110.1569) (271.1471, 110.0347) (271.1893, 109.9428) (271.2173, 109.8815) (271.2313, 109.8508) knots 0 0 0 0 0 0 0.01428571 0.02857143 0.04285714 0.05714286 0.07142857 0.08571429 0.1 0.11428571 0.12857143 0.14285714 0.15714286 0.17142857 0.18571429 0.2 0.21428571 0.22857143 0.24285714 0.25714286 0.27142857 0.28571429 0.3 0.31428571 0.32857143 0.34285714 0.35714286 0.37142857 0.38571429 0.4 0.41428571 0.42857143 0.44285714 0.45714286 0.47142857 0.48571429 0.5 0.51428571 0.52857143 0.54285714 0.55714286 0.57142857 0.58571429 0.6 0.61428571 0.62857143 0.64285714 0.65714286 0.67142857 0.68571429 0.7 0.71428571 0.72857143 0.74285714 0.75714286 0.77142857 0.78571429 0.8 0.81428571 0.82857143 0.84285714 0.85714286 0.87142857 0.88571429 0.9 0.91428571 0.92857143 0.94285714 0.95714286 0.97142857 0.98571429 1 1 1 1 1 1
  line L4583 (264.6423, 118.8885) -> (264.6688, 118.8728) construction
  line L4584 (264.6688, 118.8728) -> (264.7215, 118.8406) construction
  line L4585 (264.7215, 118.8406) -> (264.7992, 118.7903) construction
  line L4586 (264.7992, 118.7903) -> (264.9001, 118.7193) construction
  line L4587 (264.9001, 118.7193) -> (265.0226, 118.6252) construction
  line L4588 (265.0226, 118.6252) -> (265.1426, 118.5273) construction
  line L4589 (265.1426, 118.5273) -> (265.2609, 118.4271) construction
  line L4590 (265.2609, 118.4271) -> (265.3784, 118.3256) construction
  line L4591 (265.3784, 118.3256) -> (265.4954, 118.2233) construction
  line L4592 (265.4954, 118.2233) -> (265.6117, 118.12) construction
  line L4593 (265.6117, 118.12) -> (265.7271, 118.0156) construction
  line L4594 (265.7271, 118.0156) -> (265.8414, 117.9097) construction
  line L4595 (265.8414, 117.9097) -> (265.9544, 117.8019) construction
  line L4596 (265.9544, 117.8019) -> (266.066, 117.6923) construction
  line L4597 (266.066, 117.6923) -> (266.1764, 117.581) construction
  line L4598 (266.1764, 117.581) -> (266.2857, 117.4684) construction
  line L4599 (266.2857, 117.4684) -> (266.3942, 117.3545) construction
  line L4600 (266.3942, 117.3545) -> (266.5018, 117.2397) construction
  line L4601 (266.5018, 117.2397) -> (266.6087, 117.124) construction
  line L4602 (266.6087, 117.124) -> (266.7148, 117.0073) construction
  line L4603 (266.7148, 117.0073) -> (266.8201, 116.8895) construction
  line L4604 (266.8201, 116.8895) -> (266.9246, 116.7708) construction
  line L4605 (266.9246, 116.7708) -> (267.0281, 116.6509) construction
  line L4606 (267.0281, 116.6509) -> (267.1308, 116.53) construction
  line L4607 (267.1308, 116.53) -> (267.2327, 116.4081) construction
  line L4608 (267.2327, 116.4081) -> (267.3337, 116.2852) construction
  line L4609 (267.3337, 116.2852) -> (267.434, 116.1614) construction
  line L4610 (267.434, 116.1614) -> (267.5335, 116.0367) construction
  line L4611 (267.5335, 116.0367) -> (267.6323, 115.9112) construction
  line L4612 (267.6323, 115.9112) -> (267.7304, 115.7849) construction
  line L4613 (267.7304, 115.7849) -> (267.8277, 115.6577) construction
  line L4614 (267.8277, 115.6577) -> (267.9243, 115.5297) construction
  line L4615 (267.9243, 115.5297) -> (268.0201, 115.4009) construction
  line L4616 (268.0201, 115.4009) -> (268.1152, 115.2712) construction
  line L4617 (268.1152, 115.2712) -> (268.2096, 115.1408) construction
  line L4618 (268.2096, 115.1408) -> (268.3032, 115.0095) construction
  line L4619 (268.3032, 115.0095) -> (268.3962, 114.8776) construction
  line L4620 (268.3962, 114.8776) -> (268.4884, 114.7448) construction
  line L4621 (268.4884, 114.7448) -> (268.58, 114.6114) construction
  line L4622 (268.58, 114.6114) -> (268.6708, 114.4772) construction
  line L4623 (268.6708, 114.4772) -> (268.761, 114.3423) construction
  line L4624 (268.761, 114.3423) -> (268.8505, 114.2067) construction
  line L4625 (268.8505, 114.2067) -> (268.9393, 114.0705) construction
  line L4626 (268.9393, 114.0705) -> (269.0275, 113.9335) construction
  line L4627 (269.0275, 113.9335) -> (269.1149, 113.7958) construction
  line L4628 (269.1149, 113.7958) -> (269.2017, 113.6575) construction
  line L4629 (269.2017, 113.6575) -> (269.2878, 113.5185) construction
  line L4630 (269.2878, 113.5185) -> (269.3733, 113.3789) construction
  line L4631 (269.3733, 113.3789) -> (269.4581, 113.2386) construction
  line L4632 (269.4581, 113.2386) -> (269.5422, 113.0977) construction
  line L4633 (269.5422, 113.0977) -> (269.6257, 112.9562) construction
  line L4634 (269.6257, 112.9562) -> (269.7085, 112.814) construction
  line L4635 (269.7085, 112.814) -> (269.7907, 112.6712) construction
  line L4636 (269.7907, 112.6712) -> (269.8723, 112.5279) construction
  line L4637 (269.8723, 112.5279) -> (269.9532, 112.3839) construction
  line L4638 (269.9532, 112.3839) -> (270.0334, 112.2393) construction
  line L4639 (270.0334, 112.2393) -> (270.113, 112.0942) construction
  line L4640 (270.113, 112.0942) -> (270.192, 111.9485) construction
  line L4641 (270.192, 111.9485) -> (270.2703, 111.8022) construction
  line L4642 (270.2703, 111.8022) -> (270.348, 111.6553) construction
  line L4643 (270.348, 111.6553) -> (270.4251, 111.5079) construction
  line L4644 (270.4251, 111.5079) -> (270.5015, 111.3599) construction
  line L4645 (270.5015, 111.3599) -> (270.5773, 111.2114) construction
  line L4646 (270.5773, 111.2114) -> (270.6525, 111.0623) construction
  line L4647 (270.6525, 111.0623) -> (270.727, 110.9127) construction
  line L4648 (270.727, 110.9127) -> (270.801, 110.7626) construction
  line L4649 (270.801, 110.7626) -> (270.8743, 110.6119) construction
  line L4650 (270.8743, 110.6119) -> (270.9469, 110.4607) construction
  line L4651 (270.9469, 110.4607) -> (271.019, 110.3091) construction
  line L4652 (271.019, 110.3091) -> (271.0904, 110.1569) construction
  line L4653 (271.0904, 110.1569) -> (271.1471, 110.0347) construction
  line L4654 (271.1471, 110.0347) -> (271.1893, 109.9428) construction
  line L4655 (271.1893, 109.9428) -> (271.2173, 109.8815) construction
  line L4656 (271.2173, 109.8815) -> (271.2313, 109.8508) construction
  spline S62 degree 5 poles (268.1665, 125.8052) (268.1948, 125.7929) (268.2518, 125.7692) (268.3382, 125.736) (268.4549, 125.6961) (268.6031, 125.6522) (268.7528, 125.6127) (268.9034, 125.5759) (269.0546, 125.5405) (269.2061, 125.506) (269.358, 125.4726) (269.5103, 125.4406) (269.6632, 125.4104) (269.8168, 125.3824) (269.9711, 125.3565) (270.126, 125.3326) (270.2814, 125.3103) (270.4372, 125.2895) (270.5934, 125.2699) (270.7499, 125.2515) (270.9067, 125.2342) (271.0638, 125.2182) (271.2213, 125.2035) (271.3791, 125.1902) (271.5373, 125.1782) (271.6958, 125.1675) (271.8546, 125.158) (272.0137, 125.1496) (272.1731, 125.1423) (272.3327, 125.1362) (272.4925, 125.1311) (272.6526, 125.1271) (272.8129, 125.1243) (272.9735, 125.1224) (273.1343, 125.1217) (273.2953, 125.122) (273.4565, 125.1234) (273.6179, 125.1258) (273.7795, 125.1292) (273.9413, 125.1335) (274.1032, 125.1389) (274.2654, 125.1452) (274.4277, 125.1525) (274.5901, 125.1608) (274.7527, 125.17) (274.9155, 125.1801) (275.0784, 125.1912) (275.2415, 125.2033) (275.4047, 125.2162) (275.568, 125.23) (275.7315, 125.2448) (275.8951, 125.2604) (276.0588, 125.277) (276.2226, 125.2944) (276.3865, 125.3127) (276.5505, 125.3319) (276.7146, 125.352) (276.8788, 125.3729) (277.0431, 125.3946) (277.2075, 125.4172) (277.372, 125.4407) (277.5366, 125.465) (277.7012, 125.4902) (277.866, 125.5161) (278.0307, 125.5429) (278.1956, 125.5706) (278.3605, 125.599) (278.5255, 125.6282) (278.6905, 125.6583) (278.8556, 125.6892) (279.0207, 125.7208) (279.1528, 125.7468) (279.2519, 125.7666) (279.318, 125.78) (279.3511, 125.7868) knots 0 0 0 0 0 0 0.01428571 0.02857143 0.04285714 0.05714286 0.07142857 0.08571429 0.1 0.11428571 0.12857143 0.14285714 0.15714286 0.17142857 0.18571429 0.2 0.21428571 0.22857143 0.24285714 0.25714286 0.27142857 0.28571429 0.3 0.31428571 0.32857143 0.34285714 0.35714286 0.37142857 0.38571429 0.4 0.41428571 0.42857143 0.44285714 0.45714286 0.47142857 0.48571429 0.5 0.51428571 0.52857143 0.54285714 0.55714286 0.57142857 0.58571429 0.6 0.61428571 0.62857143 0.64285714 0.65714286 0.67142857 0.68571429 0.7 0.71428571 0.72857143 0.74285714 0.75714286 0.77142857 0.78571429 0.8 0.81428571 0.82857143 0.84285714 0.85714286 0.87142857 0.88571429 0.9 0.91428571 0.92857143 0.94285714 0.95714286 0.97142857 0.98571429 1 1 1 1 1 1
  line L4657 (268.1665, 125.8052) -> (268.1948, 125.7929) construction
  line L4658 (268.1948, 125.7929) -> (268.2518, 125.7692) construction
  line L4659 (268.2518, 125.7692) -> (268.3382, 125.736) construction
  line L4660 (268.3382, 125.736) -> (268.4549, 125.6961) construction
  line L4661 (268.4549, 125.6961) -> (268.6031, 125.6522) construction
  line L4662 (268.6031, 125.6522) -> (268.7528, 125.6127) construction
  line L4663 (268.7528, 125.6127) -> (268.9034, 125.5759) construction
  line L4664 (268.9034, 125.5759) -> (269.0546, 125.5405) construction
  line L4665 (269.0546, 125.5405) -> (269.2061, 125.506) construction
  line L4666 (269.2061, 125.506) -> (269.358, 125.4726) construction
  line L4667 (269.358, 125.4726) -> (269.5103, 125.4406) construction
  line L4668 (269.5103, 125.4406) -> (269.6632, 125.4104) construction
  line L4669 (269.6632, 125.4104) -> (269.8168, 125.3824) construction
  line L4670 (269.8168, 125.3824) -> (269.9711, 125.3565) construction
  line L4671 (269.9711, 125.3565) -> (270.126, 125.3326) construction
  line L4672 (270.126, 125.3326) -> (270.2814, 125.3103) construction
  line L4673 (270.2814, 125.3103) -> (270.4372, 125.2895) construction
  line L4674 (270.4372, 125.2895) -> (270.5934, 125.2699) construction
  line L4675 (270.5934, 125.2699) -> (270.7499, 125.2515) construction
  line L4676 (270.7499, 125.2515) -> (270.9067, 125.2342) construction
  line L4677 (270.9067, 125.2342) -> (271.0638, 125.2182) construction
  line L4678 (271.0638, 125.2182) -> (271.2213, 125.2035) construction
  line L4679 (271.2213, 125.2035) -> (271.3791, 125.1902) construction
  line L4680 (271.3791, 125.1902) -> (271.5373, 125.1782) construction
  line L4681 (271.5373, 125.1782) -> (271.6958, 125.1675) construction
  line L4682 (271.6958, 125.1675) -> (271.8546, 125.158) construction
  line L4683 (271.8546, 125.158) -> (272.0137, 125.1496) construction
  line L4684 (272.0137, 125.1496) -> (272.1731, 125.1423) construction
  line L4685 (272.1731, 125.1423) -> (272.3327, 125.1362) construction
  line L4686 (272.3327, 125.1362) -> (272.4925, 125.1311) construction
  line L4687 (272.4925, 125.1311) -> (272.6526, 125.1271) construction
  line L4688 (272.6526, 125.1271) -> (272.8129, 125.1243) construction
  line L4689 (272.8129, 125.1243) -> (272.9735, 125.1224) construction
  line L4690 (272.9735, 125.1224) -> (273.1343, 125.1217) construction
  line L4691 (273.1343, 125.1217) -> (273.2953, 125.122) construction
  line L4692 (273.2953, 125.122) -> (273.4565, 125.1234) construction
  line L4693 (273.4565, 125.1234) -> (273.6179, 125.1258) construction
  line L4694 (273.6179, 125.1258) -> (273.7795, 125.1292) construction
  line L4695 (273.7795, 125.1292) -> (273.9413, 125.1335) construction
  line L4696 (273.9413, 125.1335) -> (274.1032, 125.1389) construction
  line L4697 (274.1032, 125.1389) -> (274.2654, 125.1452) construction
  line L4698 (274.2654, 125.1452) -> (274.4277, 125.1525) construction
  line L4699 (274.4277, 125.1525) -> (274.5901, 125.1608) construction
  line L4700 (274.5901, 125.1608) -> (274.7527, 125.17) construction
  line L4701 (274.7527, 125.17) -> (274.9155, 125.1801) construction
  line L4702 (274.9155, 125.1801) -> (275.0784, 125.1912) construction
  line L4703 (275.0784, 125.1912) -> (275.2415, 125.2033) construction
  line L4704 (275.2415, 125.2033) -> (275.4047, 125.2162) construction
  line L4705 (275.4047, 125.2162) -> (275.568, 125.23) construction
  line L4706 (275.568, 125.23) -> (275.7315, 125.2448) construction
  line L4707 (275.7315, 125.2448) -> (275.8951, 125.2604) construction
  line L4708 (275.8951, 125.2604) -> (276.0588, 125.277) construction
  line L4709 (276.0588, 125.277) -> (276.2226, 125.2944) construction
  line L4710 (276.2226, 125.2944) -> (276.3865, 125.3127) construction
  line L4711 (276.3865, 125.3127) -> (276.5505, 125.3319) construction
  line L4712 (276.5505, 125.3319) -> (276.7146, 125.352) construction
  line L4713 (276.7146, 125.352) -> (276.8788, 125.3729) construction
  line L4714 (276.8788, 125.3729) -> (277.0431, 125.3946) construction
  line L4715 (277.0431, 125.3946) -> (277.2075, 125.4172) construction
  line L4716 (277.2075, 125.4172) -> (277.372, 125.4407) construction
  line L4717 (277.372, 125.4407) -> (277.5366, 125.465) construction
  line L4718 (277.5366, 125.465) -> (277.7012, 125.4902) construction
  line L4719 (277.7012, 125.4902) -> (277.866, 125.5161) construction
  line L4720 (277.866, 125.5161) -> (278.0307, 125.5429) construction
  line L4721 (278.0307, 125.5429) -> (278.1956, 125.5706) construction
  line L4722 (278.1956, 125.5706) -> (278.3605, 125.599) construction
  line L4723 (278.3605, 125.599) -> (278.5255, 125.6282) construction
  line L4724 (278.5255, 125.6282) -> (278.6905, 125.6583) construction
  line L4725 (278.6905, 125.6583) -> (278.8556, 125.6892) construction
  line L4726 (278.8556, 125.6892) -> (279.0207, 125.7208) construction
  line L4727 (279.0207, 125.7208) -> (279.1528, 125.7468) construction
  line L4728 (279.1528, 125.7468) -> (279.2519, 125.7666) construction
  line L4729 (279.2519, 125.7666) -> (279.318, 125.78) construction
  line L4730 (279.318, 125.78) -> (279.3511, 125.7868) construction
  arc A125 (214.3883, 221.4115) -> (209.8757, 221.4115) centre (212.132, 150) ccw
  arc A126 (283.5435, 147.7437) -> (283.5435, 152.2563) centre (212.132, 150) ccw
  arc A127 (279.3511, 125.7868) -> (280.7456, 130.0785) centre (212.132, 150) ccw
  spline S63 degree 5 poles (181.0205, 202.5103) (181.0048, 202.5368) (180.9726, 202.5895) (180.9223, 202.6672) (180.8513, 202.7681) (180.7572, 202.8906) (180.6593, 203.0106) (180.5591, 203.1289) (180.4576, 203.2464) (180.3553, 203.3634) (180.252, 203.4797) (180.1476, 203.5951) (180.0417, 203.7094) (179.9339, 203.8224) (179.8243, 203.934) (179.713, 204.0444) (179.6004, 204.1537) (179.4865, 204.2622) (179.3717, 204.3698) (179.256, 204.4767) (179.1393, 204.5828) (179.0215, 204.6881) (178.9028, 204.7926) (178.7829, 204.8961) (178.662, 204.9988) (178.5401, 205.1007) (178.4172, 205.2017) (178.2934, 205.302) (178.1687, 205.4015) (178.0432, 205.5003) (177.9169, 205.5984) (177.7897, 205.6957) (177.6617, 205.7923) (177.5329, 205.8881) (177.4032, 205.9832) (177.2728, 206.0776) (177.1415, 206.1712) (177.0096, 206.2642) (176.8768, 206.3564) (176.7434, 206.448) (176.6092, 206.5388) (176.4743, 206.629) (176.3387, 206.7185) (176.2025, 206.8073) (176.0655, 206.8955) (175.9278, 206.9829) (175.7895, 207.0697) (175.6505, 207.1558) (175.5109, 207.2413) (175.3706, 207.3261) (175.2297, 207.4102) (175.0882, 207.4937) (174.946, 207.5765) (174.8032, 207.6587) (174.6599, 207.7403) (174.5159, 207.8212) (174.3713, 207.9014) (174.2262, 207.981) (174.0805, 208.06) (173.9342, 208.1383) (173.7873, 208.216) (173.6399, 208.2931) (173.4919, 208.3695) (173.3434, 208.4453) (173.1943, 208.5205) (173.0447, 208.595) (172.8946, 208.669) (172.7439, 208.7423) (172.5927, 208.8149) (172.4411, 208.887) (172.2889, 208.9584) (172.1667, 209.0151) (172.0748, 209.0573) (172.0135, 209.0853) (171.9828, 209.0993) knots 0 0 0 0 0 0 0.01428571 0.02857143 0.04285714 0.05714286 0.07142857 0.08571429 0.1 0.11428571 0.12857143 0.14285714 0.15714286 0.17142857 0.18571429 0.2 0.21428571 0.22857143 0.24285714 0.25714286 0.27142857 0.28571429 0.3 0.31428571 0.32857143 0.34285714 0.35714286 0.37142857 0.38571429 0.4 0.41428571 0.42857143 0.44285714 0.45714286 0.47142857 0.48571429 0.5 0.51428571 0.52857143 0.54285714 0.55714286 0.57142857 0.58571429 0.6 0.61428571 0.62857143 0.64285714 0.65714286 0.67142857 0.68571429 0.7 0.71428571 0.72857143 0.74285714 0.75714286 0.77142857 0.78571429 0.8 0.81428571 0.82857143 0.84285714 0.85714286 0.87142857 0.88571429 0.9 0.91428571 0.92857143 0.94285714 0.95714286 0.97142857 0.98571429 1 1 1 1 1 1
  line L4731 (181.0205, 202.5103) -> (181.0048, 202.5368) construction
  line L4732 (181.0048, 202.5368) -> (180.9726, 202.5895) construction
  line L4733 (180.9726, 202.5895) -> (180.9223, 202.6672) construction
  line L4734 (180.9223, 202.6672) -> (180.8513, 202.7681) construction
  line L4735 (180.8513, 202.7681) -> (180.7572, 202.8906) construction
  line L4736 (180.7572, 202.8906) -> (180.6593, 203.0106) construction
  line L4737 (180.6593, 203.0106) -> (180.5591, 203.1289) construction
  line L4738 (180.5591, 203.1289) -> (180.4576, 203.2464) construction
  line L4739 (180.4576, 203.2464) -> (180.3553, 203.3634) construction
  line L4740 (180.3553, 203.3634) -> (180.252, 203.4797) construction
  line L4741 (180.252, 203.4797) -> (180.1476, 203.5951) construction
  line L4742 (180.1476, 203.5951) -> (180.0417, 203.7094) construction
  line L4743 (180.0417, 203.7094) -> (179.9339, 203.8224) construction
  line L4744 (179.9339, 203.8224) -> (179.8243, 203.934) construction
  line L4745 (179.8243, 203.934) -> (179.713, 204.0444) construction
  line L4746 (179.713, 204.0444) -> (179.6004, 204.1537) construction
  line L4747 (179.6004, 204.1537) -> (179.4865, 204.2622) construction
  line L4748 (179.4865, 204.2622) -> (179.3717, 204.3698) construction
  line L4749 (179.3717, 204.3698) -> (179.256, 204.4767) construction
  line L4750 (179.256, 204.4767) -> (179.1393, 204.5828) construction
  line L4751 (179.1393, 204.5828) -> (179.0215, 204.6881) construction
  line L4752 (179.0215, 204.6881) -> (178.9028, 204.7926) construction
  line L4753 (178.9028, 204.7926) -> (178.7829, 204.8961) construction
  line L4754 (178.7829, 204.8961) -> (178.662, 204.9988) construction
  line L4755 (178.662, 204.9988) -> (178.5401, 205.1007) construction
  line L4756 (178.5401, 205.1007) -> (178.4172, 205.2017) construction
  line L4757 (178.4172, 205.2017) -> (178.2934, 205.302) construction
  line L4758 (178.2934, 205.302) -> (178.1687, 205.4015) construction
  line L4759 (178.1687, 205.4015) -> (178.0432, 205.5003) construction
  line L4760 (178.0432, 205.5003) -> (177.9169, 205.5984) construction
  line L4761 (177.9169, 205.5984) -> (177.7897, 205.6957) construction
  line L4762 (177.7897, 205.6957) -> (177.6617, 205.7923) construction
  line L4763 (177.6617, 205.7923) -> (177.5329, 205.8881) construction
  line L4764 (177.5329, 205.8881) -> (177.4032, 205.9832) construction
  line L4765 (177.4032, 205.9832) -> (177.2728, 206.0776) construction
  line L4766 (177.2728, 206.0776) -> (177.1415, 206.1712) construction